Autodesk Inventor part; units mm, degrees
(part 2 of 2)
sketch "Sketch23" plane through (0, 6.35, 0) normal (0, 1, 0) x (1, 0, 0)
  line L0 (420.6633, 458.2268) -> (433.3633, 458.2268)
  line L1 (433.3633, 458.2268) -> (433.3633, 445.5268)
  line L2 (433.3633, 445.5268) -> (420.6633, 445.5268)
  line L3 (420.6633, 445.5268) -> (420.6633, 458.2268)
  line L4 (-74.6367, 451.8768) -> (-61.9367, 451.8768)
  line L5 (-61.9367, 451.8768) -> (-61.9367, 458.2268)
  line L6 (-61.9367, 458.2268) -> (-74.6367, 458.2268)
  line L7 (-74.6367, 458.2268) -> (-74.6367, 451.8768)
  point P0 (0, 0)
  dimension "d187" = 12.7
  dimension "d188" = 12.7
  constraints: 16 end point, 4 parallel, 2 horizontal, 2 perpendicular
  measures "d187" distance of L0.end L1.end
  measures "d188" distance of L6.end L5.end
extrude "Extrusion22" add sketch "Sketch23" against normal blind 6.35
sketch "Sketch24" plane through (0, 6.35, 0) normal (0, 1, 0) x (1, 0, 0)
  line L0 (-74.6367, 458.2268) -> (-74.6367, 289.3168) projected
  line L1 (-74.6367, 445.5268) -> (-68.2867, 445.5268)
  line L2 (-68.2867, 445.5268) -> (-68.2867, 420.1268)
  line L3 (-68.2867, 420.1268) -> (-74.6367, 420.1268)
  line L4 (-74.6367, 420.1268) -> (-74.6367, 445.5268)
  line L5 (-68.2867, 420.1268) -> (-74.6367, 420.1268)
  line L6 (-74.6367, 420.1268) -> (-74.6367, 394.7268)
  line L7 (-74.6367, 394.7268) -> (-68.2867, 394.7268)
  line L8 (-68.2867, 394.7268) -> (-68.2867, 420.1268)
  line L9 (-68.2867, 394.7268) -> (-74.6367, 394.7268)
  line L10 (-74.6367, 394.7268) -> (-74.6367, 343.9268)
  line L11 (-74.6367, 343.9268) -> (-68.2867, 343.9268)
  line L12 (-68.2867, 343.9268) -> (-68.2867, 394.7268)
  line L13 (-68.2867, 343.9268) -> (-74.6367, 343.9268)
  line L14 (-74.6367, 343.9268) -> (-74.6367, 318.5268)
  line L15 (-74.6367, 318.5268) -> (-68.2867, 318.5268)
  line L16 (-68.2867, 318.5268) -> (-68.2867, 343.9268)
  line L17 (-68.2867, 318.5268) -> (-74.6367, 318.5268)
  line L18 (-74.6367, 318.5268) -> (-74.6367, 289.3168)
  line L19 (-74.6367, 289.3168) -> (-68.2867, 289.3168)
  line L20 (-68.2867, 289.3168) -> (-68.2867, 318.5268)
  point P0 (0, 0)
  constraints: 40 end point, 10 parallel, 5 horizontal, 5 perpendicular, 4 point on line
extrude "Extrusion23" cut sketch "Sketch24" against normal blind 6.35 contours L1 L2 L3 L0 | L7 L12 L11 L0 | L15 L20 L19 L0
sketch "Sketch25" plane through (0, 6.35, 0) normal (0, 1, 0) x (1, 0, 0)
  line L0 (-68.2867, 318.5268) -> (-68.2867, 119.1368) projected
  line L1 (-68.2867, 318.5268) -> (-74.6367, 318.5268)
  line L2 (-74.6367, 318.5268) -> (-74.6367, 267.7268)
  line L3 (-74.6367, 267.7268) -> (-68.2867, 267.7268)
  line L4 (-68.2867, 267.7268) -> (-68.2867, 318.5268)
  line L5 (-68.2867, 267.7268) -> (-74.6367, 267.7268)
  line L6 (-74.6367, 267.7268) -> (-74.6367, 242.3268)
  line L7 (-74.6367, 242.3268) -> (-68.2867, 242.3268)
  line L8 (-68.2867, 242.3268) -> (-68.2867, 267.7268)
  line L9 (-68.2867, 242.3268) -> (-74.6367, 242.3268)
  line L10 (-74.6367, 242.3268) -> (-74.6367, 191.5268)
  line L11 (-74.6367, 191.5268) -> (-68.2867, 191.5268)
  line L12 (-68.2867, 191.5268) -> (-68.2867, 242.3268)
  line L13 (-74.6367, 191.5268) -> (-68.2867, 191.5268)
  line L14 (-68.2867, 191.5268) -> (-68.2867, 166.1268)
  line L15 (-68.2867, 166.1268) -> (-74.6367, 166.1268)
  line L16 (-74.6367, 166.1268) -> (-74.6367, 191.5268)
  point P0 (0, 0)
  constraints: 32 end point, 8 parallel, 4 horizontal, 4 perpendicular, 1 point on line
extrude "Extrusion24" add sketch "Sketch25" against normal blind 6.35 contours L0 L7 L6 L3 | L0 L15 L16 L11
sketch "Sketch26" plane through (0, 6.35, 0) normal (0, 1, 0) x (1, 0, 0)
  line L0 (20.6133, 350.2308) -> (20.6133, 58.2229) projected
  line L1 (338.1133, 58.2229) -> (338.1133, 350.2308) projected
  line L2 (-68.2867, 119.1368) -> (-42.8867, 119.1368)
  line L3 (-42.8867, 119.1368) -> (-42.8867, 125.4868)
  line L4 (-42.8867, 125.4868) -> (-68.2867, 125.4868)
  line L5 (-68.2867, 125.4868) -> (-68.2867, 119.1368)
  line L6 (-42.8867, 125.4868) -> (-17.4867, 125.4868)
  line L7 (-17.4867, 125.4868) -> (-17.4867, 119.1368)
  line L8 (-17.4867, 119.1368) -> (-42.8867, 119.1368)
  line L9 (-42.8867, 119.1368) -> (-42.8867, 125.4868)
  line L10 (427.0133, 119.1368) -> (401.6133, 119.1368)
  line L11 (401.6133, 119.1368) -> (401.6133, 125.4868)
  line L12 (401.6133, 125.4868) -> (427.0133, 125.4868)
  line L13 (427.0133, 125.4868) -> (427.0133, 119.1368)
  line L14 (401.6133, 125.4868) -> (376.2133, 125.4868)
  line L15 (376.2133, 125.4868) -> (376.2133, 119.1368)
  line L16 (376.2133, 119.1368) -> (401.6133, 119.1368)
  line L17 (401.6133, 119.1368) -> (401.6133, 125.4868)
  line L18 (338.1133, 125.4868) -> (293.6633, 125.4868)
  line L19 (293.6633, 125.4868) -> (293.6633, 119.1368)
  line L20 (293.6633, 119.1368) -> (338.1133, 119.1368)
  line L21 (338.1133, 119.1368) -> (338.1133, 125.4868)
  line L22 (293.6633, 125.4868) -> (268.2633, 125.4868)
  line L23 (268.2633, 125.4868) -> (268.2633, 119.1368)
  line L24 (268.2633, 119.1368) -> (293.6633, 119.1368)
  line L25 (293.6633, 119.1368) -> (293.6633, 125.4868)
  line L26 (20.6133, 125.4868) -> (65.0633, 125.4868)
  line L27 (65.0633, 125.4868) -> (65.0633, 119.1368)
  line L28 (65.0633, 119.1368) -> (20.6133, 119.1368)
  line L29 (20.6133, 119.1368) -> (20.6133, 125.4868)
  line L30 (65.0633, 125.4868) -> (90.4633, 125.4868)
  line L31 (90.4633, 125.4868) -> (90.4633, 119.1368)
  line L32 (90.4633, 119.1368) -> (65.0633, 119.1368)
  line L33 (65.0633, 119.1368) -> (65.0633, 125.4868)
  line L34 (90.4633, 125.4868) -> (166.6633, 125.4868)
  line L35 (166.6633, 125.4868) -> (166.6633, 119.1368)
  line L36 (166.6633, 119.1368) -> (90.4633, 119.1368)
  line L37 (90.4633, 119.1368) -> (90.4633, 125.4868)
  line L38 (166.6633, 125.4868) -> (192.0633, 125.4868)
  line L39 (192.0633, 125.4868) -> (192.0633, 119.1368)
  line L40 (192.0633, 119.1368) -> (166.6633, 119.1368)
  line L41 (166.6633, 119.1368) -> (166.6633, 125.4868)
  point P0 (0, 0)
  dimension "d195" = 25.4
  dimension "d196" = 6.35
  dimension "d197" = 25.4
  dimension "d198" = 25.4
  dimension "d199" = 25.4
  dimension "d200" = 44.45
  dimension "d201" = 25.4
  dimension "d202" = 44.45
  dimension "d203" = 25.4
  dimension "d204" = 76.2
  dimension "d205" = 25.4
  constraints: 80 end point, 20 parallel, 10 horizontal, 10 perpendicular, 4 point on line
  measures "d195" distance of L4.end L3.end
  measures "d196" distance of L3.end L2.end
  measures "d197" distance of L7.end L8.end
  measures "d198" distance of L11.end L12.end
  measures "d199" distance of L16.end L15.end
  measures "d200" distance of L20.end L19.end
  measures "d201" distance of L24.end L23.end
  measures "d202" distance of L27.end L28.end
  measures "d203" distance of L31.end L32.end
  measures "d204" distance of L35.end L36.end
  measures "d205" distance of L39.end L40.end
extrude "Extrusion25" cut sketch "Sketch26" against normal blind 6.35 contours L30 L31 L32 L27 | L38 L39 L40 L35 | L24 L23 L22 L19 | L3 L6 L7 L8 | L16 L15 L14 L11
sketch "Sketch27" plane through (0, 6.35, 0) normal (0, 1, 0) x (1, 0, 0)
  line L0 (90.4633, 119.1368) -> (65.0633, 119.1368) projected
  line L1 (65.0633, 119.1368) -> (65.0633, 125.4868) projected
  line L2 (65.0633, 125.4868) -> (90.4633, 125.4868) projected
  line L3 (90.4633, 125.4868) -> (90.4633, 119.1368) projected
  line L4 (268.2633, 119.1368) -> (268.2633, 125.4868) projected
  line L5 (268.2633, 125.4868) -> (293.6633, 125.4868) projected
  line L6 (293.6633, 125.4868) -> (293.6633, 119.1368) projected
  line L7 (293.6633, 119.1368) -> (268.2633, 119.1368) projected
  line L8 (166.6633, 125.4868) -> (192.0633, 125.4868) projected
  line L9 (65.0633, 125.4868) -> (52.3633, 125.4868)
  line L10 (52.3633, 125.4868) -> (52.3633, 119.1368)
  line L11 (52.3633, 119.1368) -> (65.0633, 119.1368)
  line L12 (65.0633, 119.1368) -> (65.0633, 125.4868)
  line L13 (52.3633, 125.4868) -> (103.1633, 125.4868)
  line L14 (103.1633, 125.4868) -> (103.1633, 119.1368)
  line L15 (103.1633, 119.1368) -> (52.3633, 119.1368)
  line L16 (52.3633, 119.1368) -> (52.3633, 125.4868)
  line L17 (268.2633, 125.4868) -> (255.5633, 125.4868)
  line L18 (255.5633, 125.4868) -> (255.5633, 119.1368)
  line L19 (255.5633, 119.1368) -> (268.2633, 119.1368)
  line L20 (268.2633, 119.1368) -> (268.2633, 125.4868)
  line L21 (255.5633, 119.1368) -> (306.3633, 119.1368)
  line L22 (306.3633, 119.1368) -> (306.3633, 125.4868)
  line L23 (306.3633, 125.4868) -> (255.5633, 125.4868)
  line L24 (255.5633, 125.4868) -> (255.5633, 119.1368)
  point P0 (0, 0)
  dimension "d208" = 12.7
  dimension "d209" = 50.8
  dimension "d210" = 12.7
  dimension "d211" = 50.8
  constraints: 32 end point, 8 parallel, 4 horizontal, 4 perpendicular, 1 point on line
  measures "d208" distance of L11.end L10.end
  measures "d209" distance of L14.end L15.end
  measures "d210" distance of L19.end L18.end
  measures "d211" distance of L23.end L22.end
extrude "Extrusion26" cut sketch "Sketch27" against normal blind 6.35 contours L3 L13 L14 L15 | L11 L10 L9 L1 | L19 L18 L17 L4 | L6 L23 L22 L21
sketch "Sketch28" plane through (0, 6.35, 0) normal (0, 1, 0) x (1, 0, 0)
  circle A0 centre (54.6239, -1.2338) radius 1.9812 projected
  circle A1 centre (-26.0973, 79.4874) radius 1.9812 projected
  circle A2 centre (54.6239, 79.4874) radius 1.9812 projected
  circle A3 centre (-26.0973, -1.2338) radius 1.9812 projected
  point P0 (0, 0)
extrude "Extrusion27" add sketch "Sketch28" against normal blind 6.35
sketch "Sketch29" plane through (0, 6.35, 0) normal (0, 1, 0) x (1, 0, 0)
  circle A0 centre (-26.0973, 409.6874) radius 1.9812 projected
  circle A1 centre (-26.0973, 328.9662) radius 1.9812 projected
  circle A2 centre (54.6239, 409.6874) radius 1.9812 projected
  circle A3 centre (54.6239, 328.9662) radius 1.9812 projected
  point P0 (0, 0)
extrude "Extrusion28" add sketch "Sketch29" against normal blind 6.35
sketch "Sketch30" plane through (0, 6.35, 0) normal (0, 1, 0) x (1, 0, 0)
  circle A0 centre (304.1027, 79.4874) radius 1.9812 projected
  circle A1 centre (384.8239, 79.4874) radius 1.9812 projected
  circle A2 centre (304.1027, 409.6874) radius 1.9812 projected
  circle A3 centre (384.8239, -1.2338) radius 1.9812 projected
  circle A4 centre (304.1027, 328.9662) radius 1.9812 projected
  circle A5 centre (304.1027, -1.2338) radius 1.9812 projected
  circle A6 centre (384.8239, 328.9662) radius 1.9812 projected
  circle A7 centre (384.8239, 409.6874) radius 1.9812 projected
  point P0 (0, 0)
extrude "Extrusion29" add sketch "Sketch30" against normal blind 6.35
sketch "Sketch31" plane through (0, 6.35, 0) normal (0, 1, 0) x (1, 0, 0)
  arc A0 (334.9383, 55.6246) -> (353.9883, 55.6246) centre (344.4633, 39.1268) ccw projected
  arc A1 (23.7883, 352.829) -> (4.7383, 352.829) centre (14.2633, 369.3268) ccw projected
  line L0 (344.4633, 39.1268) -> (303.9757, 39.1268)
  line L1 (303.9757, 39.1268) -> (303.9757, -1.3608)
  line L2 (303.9757, -1.3608) -> (344.4633, -1.3608)
  line L3 (344.4633, -1.3608) -> (344.4633, 39.1268)
  line L4 (303.9757, -1.3608) -> (384.9509, -1.3608)
  line L5 (384.9509, -1.3608) -> (384.9509, 79.6144)
  line L6 (384.9509, 79.6144) -> (303.9757, 79.6144)
  line L7 (303.9757, 79.6144) -> (303.9757, -1.3608)
  line L8 (14.2633, 369.3268) -> (-26.2243, 369.3268)
  line L9 (-26.2243, 369.3268) -> (-26.2243, 328.8392)
  line L10 (-26.2243, 328.8392) -> (14.2633, 328.8392)
  line L11 (14.2633, 328.8392) -> (14.2633, 369.3268)
  line L12 (-26.2243, 328.8392) -> (54.7509, 328.8392)
  line L13 (54.7509, 328.8392) -> (54.7509, 409.8144)
  line L14 (54.7509, 409.8144) -> (-26.2243, 409.8144)
  line L15 (-26.2243, 409.8144) -> (-26.2243, 328.8392)
  line L16 (-30.1867, -1.3608) -> (54.7509, -1.3608)
  line L17 (54.7509, -1.3608) -> (54.7509, 79.6144)
  line L18 (54.7509, 79.6144) -> (-30.1867, 79.6144)
  line L19 (-30.1867, 79.6144) -> (-30.1867, -1.3608)
  line L20 (303.9757, 328.8392) -> (384.9509, 328.8392)
  line L21 (384.9509, 328.8392) -> (384.9509, 409.8144)
  line L22 (384.9509, 409.8144) -> (303.9757, 409.8144)
  line L23 (303.9757, 409.8144) -> (303.9757, 328.8392)
  circle A2 centre (-30.1867, -1.3608) radius 1.9812
  circle A3 centre (-30.1867, 79.6144) radius 1.9812
  circle A4 centre (54.7509, 79.6144) radius 1.9812
  circle A5 centre (54.7509, -1.3608) radius 1.9812
  circle A6 centre (303.9757, -1.3608) radius 1.9812
  circle A7 centre (303.9757, 79.6144) radius 1.9812
  circle A8 centre (384.9509, 79.6144) radius 1.9812
  circle A9 centre (384.9509, -1.3608) radius 1.9812
  circle A10 centre (-26.2243, 328.8392) radius 1.9812
  circle A11 centre (-26.2243, 409.8144) radius 1.9812
  circle A12 centre (54.7509, 409.8144) radius 1.9812
  circle A13 centre (54.7509, 328.8392) radius 1.9812
  circle A14 centre (303.9757, 328.8392) radius 1.9812
  circle A15 centre (303.9757, 409.8144) radius 1.9812
  circle A16 centre (384.9509, 409.8144) radius 1.9812
  circle A17 centre (384.9509, 328.8392) radius 1.9812
  point P0 (0, 0)
  dimension "d220" = 40.4876
  dimension "d221" = 40.4876
  dimension "d222" = 80.9752
  dimension "d223" = 80.9752
  dimension "d224" = 40.4876
  dimension "d225" = 40.4876
  dimension "d226" = 80.9752
  dimension "d227" = 80.9752
  dimension "d228" = 3.9624
  dimension "d229" = 3.9624
  dimension "d230" = 3.9624
  dimension "d231" = 3.9624
  dimension "d232" = 3.9624
  dimension "d233" = 3.9624
  dimension "d234" = 3.9624
  dimension "d235" = 3.9624
  constraints: 48 end point, 16 centre point, 16 coincident, 12 parallel, 6 horizontal, 6 perpendicular
  measures "d220" distance of L2.end L1.end
  measures "d221" distance of L1.end L0.end
  measures "d222" distance of L6.end L5.end
  measures "d223" distance of L5.end L4.end
  measures "d224" distance of L10.end L9.end
  measures "d225" distance of L9.end L8.end
  measures "d226" distance of L14.end L13.end
  measures "d227" distance of L13.end L12.end
  measures "d228" diameter of A2
  measures "d229" diameter of A3
  measures "d230" diameter of A4
  measures "d231" diameter of A5
  measures "d232" diameter of A6
  measures "d233" diameter of A7
  measures "d234" diameter of A8
  measures "d235" diameter of A9
extrude "Extrusion30" cut sketch "Sketch31" against normal blind 6.35 contours A6 L2 L1 | L1 L2 A6 | A7 L6 L7 | L7 L6 A7 | A9 L5 L4 | L4 L5 A9 | A8 L5 L6 | L6 L5 A8 | A10 L9 L10 | L10 L9 A10 | A13 L13 L12 | L12 L13 A13 | A11 L14 L15 | L15 L14 A11 | A12 L14 L13 | L13 L14 A12 | L19 A2 L16 | L16 A2 L19 | A5 L17 L16 | L16 L17 A5 | A3 L18 L19 | L19 L18 A3 | A4 L18 L17 | L17 L18 A4 | L23 A14 L20 | L20 A14 L23 | A17 L21 L20 | L20 L21 A17 | A15 L22 L23 | L23 L22 A15 | A16 L22 L21 | L21 L22 A16
sketch "Sketch32" plane through (0, 6.35, 0) normal (0, 1, 0) x (1, 0, 0)
  circle A0 centre (-30.1867, -1.3608) radius 1.9812 projected
  circle A1 centre (-30.1867, 79.6144) radius 1.9812 projected
  point P0 (0, 0)
extrude "Extrusion31" add sketch "Sketch32" against normal blind 6.35
sketch "Sketch33" plane through (0, 6.35, 0) normal (0, 1, 0) x (1, 0, 0)
  circle A0 centre (54.7509, -1.3608) radius 1.9812 projected
  line L0 (54.7509, -1.3608) -> (-26.2243, -1.3608)
  line L1 (-26.2243, -1.3608) -> (-26.2243, 79.6144)
  line L2 (-26.2243, 79.6144) -> (54.7509, 79.6144)
  line L3 (54.7509, 79.6144) -> (54.7509, -1.3608)
  circle A1 centre (-26.2243, 79.6144) radius 1.9812
  circle A2 centre (-26.2243, -1.3608) radius 1.9812
  point P0 (0, 0)
  dimension "d240" = 80.9752
  constraints: 8 end point, 2 centre point, 2 coincident, 2 parallel, 1 horizontal, 1 perpendicular
  measures "d240" distance of L1.end L2.end
extrude "Extrusion32" cut sketch "Sketch33" against normal blind 6.35 contours A2 L1 L0 | L0 L1 A2 | A1 L1 L2 | L2 L1 A1
body "Solid1"
